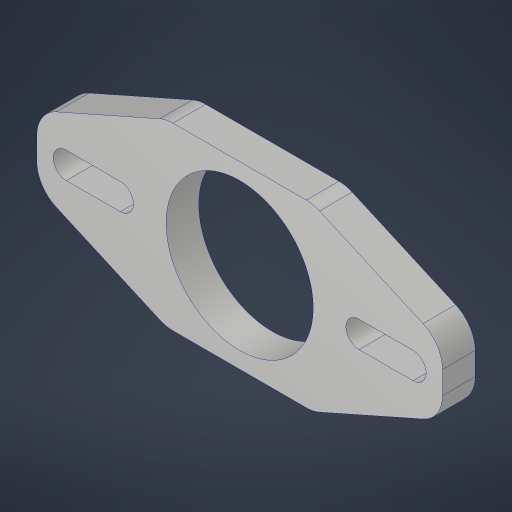
# Autodesk Inventor part: EL2-CGB-010
Saved by Autodesk Inventor 2023.4 (Build 274418000, 418)
## iProperties
Created: 2025-01-24
Part Number: EL2-CGB-010
Material: Aluminum 6061
Document SubType Name: Modeling
Designer: brand
Density: 2.7 g/cm^3
Appearance: Aluminum - Flat
Author: brand
Autodesk Inventor part; units mm, degrees
ref_plane "YZ Plane" through (0, 0, 0) normal (1, 0, 0) x (0, 1, 0)
ref_plane "XZ Plane" through (0, 0, 0) normal (0, 1, 0) x (-1, 0, 0)
sketch "Sketch1" plane through (0, 0, 0) normal (0, 0, 1) x (1, 0, 0)
  circle A0 centre (0, 0) radius 14.2875
  line L0 (-33.6677, 0) -> (-23.1902, 0) construction
  line L1 (-33.6677, -2.5527) -> (-23.1902, -2.5527)
  line L2 (-23.1902, 2.5527) -> (-33.6677, 2.5527)
  arc A1 (-33.6677, 2.5527) -> (-33.6677, -2.5527) centre (-33.6677, 0) ccw
  arc A2 (-23.1902, -2.5527) -> (-23.1902, 2.5527) centre (-23.1902, 0) ccw
  line L3 (23.1902, 0) -> (33.6677, 0) construction
  line L4 (23.1902, -2.5527) -> (33.6677, -2.5527)
  line L5 (33.6677, 2.5527) -> (23.1902, 2.5527)
  arc A3 (23.1902, 2.5527) -> (23.1902, -2.5527) centre (23.1902, 0) ccw
  arc A4 (33.6677, -2.5527) -> (33.6677, 2.5527) centre (33.6677, 0) ccw
  line L6 (-14.2875, 17.4625) -> (-39.3954, 6.35)
  line L7 (-39.3954, 6.35) -> (-39.3954, -6.35)
  line L8 (-39.3954, -6.35) -> (-14.2875, -17.4625)
  line L9 (-14.2875, -17.4625) -> (14.2875, -17.4625)
  line L10 (14.2875, -17.4625) -> (39.3954, -6.35)
  line L11 (39.3954, -6.35) -> (39.3954, 6.35)
  line L12 (39.3954, 6.35) -> (14.2875, 17.4625)
  line L13 (14.2875, 17.4625) -> (-14.2875, 17.4625)
  circle A5 centre (-23.1902, 0) radius 4.7625 construction
  circle A6 centre (0, 0) radius 13.6398 construction
  circle A7 centre (-45.9552, 70.4429) radius 54.5719 construction
  circle A8 centre (-1.8189, -39.1868) radius 18.1864 construction
  line L14 (8.4839, 74.2476) -> (16.3232, -37.9189) construction
  line L15 (-15.7788, -50.843) -> (-87.8447, 35.4663) construction
  line L16 (-45.9552, 70.4429) -> (4.7485, 67.3163) construction
  line L17 (4.7485, 67.3163) -> (-1.8189, -39.1868) construction
  point P0 (-28.429, 0)
  point P1 (28.429, 0)
  point P2 (0, 17.4625)
  point P3 (0, 14.2875)
  point P4 (-20.6375, 0)
  point P5 (-14.2875, 0)
  point P6 (-36.2204, 0)
  point P7 (-39.3954, 0)
  point P8 (39.3954, 0)
  dimension "d0" = 28.575
  dimension "d3" = 28.575
  dimension "d4" = 3.175
  dimension "d5" = 17.4625
  dimension "d6" = 17.4625
  dimension "d7" = 10.4775
  dimension "d8" = 10.4775
  dimension "d9" = 6.35
  dimension "d10" = 5.1054
  dimension "d11" = 28.429
  dimension "d12" = 9.525
  dimension "d13" = 27.2796
  dimension "d16" = 109.1438
  dimension "d19" = 36.3728
  dimension "d20" = 106.7054
  dimension "d21" = 50.8
  dimension "d22" = 28.429
  dimension "d23" = 3.175
  dimension "d24" = 5.7277
  dimension "d25" = 5.7277
  dimension "d26" = 12.7
  constraints: 40 end point, 16 point on circle, 13 tangent, 9 centre point, 6 coincident, 5 horizontal alignment, 5 midpoint, 4 perpendicular, 4 vertical alignment, 3 parallel, 2 point on line, 1 horizontal, 1 vertical
  measures "d0" diameter of A0
  measures "d3" distance of L12.end L6.start
  measures "d4" distance from line of A0.start L13
  measures "d5" distance from line of point (0, 0) L13
  measures "d6" distance from line of A0.centre L9
  measures "d7" distance of L0.start L0.end
  measures "d8" distance of L3.start L3.end
  measures "d9" distance of A0.end point (-20.637, 0)
  measures "d10" distance between parallel lines of L1 L2
  measures "d11" distance of point (0, 0) point (-28.429, 0)
  measures "d12" diameter of A5
  measures "d13" diameter of A6
  measures "d16" diameter of A7
  measures "d19" diameter of A8
  measures "d20" distance of L16.end L17.end
  measures "d21" distance of L16.start L16.end
  measures "d22" distance of point (28.429, 0) point (0, 0)
  measures "d23" distance from line of L7 point (-36.22, 0)
  measures "d24" distance from line of L7 L0.start
  measures "d25" distance from line of L11 L3.end
  measures "d26" distance of L6.end L7.end
extrude "Extrusion1" add sketch "Sketch1" along normal mid plane 6.35
fillet "Fillet1" radius 6.35 8 edges at (-14.2875, 17.4625, 0) (14.2875, 17.4625, 0) (39.3954, 6.35, 0) (39.3954, -6.35, 0) (14.2875, -17.4625, 0) (-14.2875, -17.4625, 0) (-39.3954, -6.35, 0) (-39.3954, 6.35, 0)
ref_plane "Work Plane1" through (-33.6677, 0, 3.175) normal (0, 1, 0) x (1, 0, 0)
equation "\"d6\" = d5"
body "Solid1"
